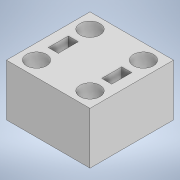
# Autodesk Inventor part: SiPM cover
Saved by Autodesk Inventor 2020 (Build 240168000, 168)
## iProperties
Created: 2021-06-25
Part Number: SiPM cover
Material: Generic
Document SubType Name: Modeling
Designer: alejandrosalazar
Density: 1 g/cm^3
Appearance: Default
Author: alejandrosalazar
Autodesk Inventor part; units mm, degrees
ref_plane "YZ Plane" through (0, 0, 0) normal (1, 0, 0) x (0, 1, 0)
ref_plane "XZ Plane" through (0, 0, 0) normal (0, 1, 0) x (-1, 0, 0)
ref_plane "XY Plane" through (0, 0, 0) normal (0, 0, 1) x (1, 0, 0)
sketch "Sketch1" plane through (0, 0, 0) normal (0, 1, 0) x (-1, 0, 0)
  line L0 (0, 0) -> (-25, 0)
  line L1 (-25, 0) -> (-25, 25)
  line L2 (-25, 25) -> (0, 25)
  line L3 (0, 25) -> (0, 0)
  line L4 (-10, 12.5) -> (-10, 15)
  line L5 (-10, 15) -> (-12.5, 15)
  line L6 (-10, 12.5) -> (-10, 10)
  line L7 (-10, 10) -> (-12.5, 10)
  line L8 (-15, 12.5) -> (-15, 15)
  line L9 (-15, 15) -> (-12.5, 15)
  line L10 (-15, 12.5) -> (-15, 10)
  line L11 (-15, 10) -> (-12.5, 10)
  circle A0 centre (-4.5, 4.5) radius 3
  circle A1 centre (-20.5, 20.5) radius 3
  circle A2 centre (-4.5, 20.5) radius 3
  circle A3 centre (-20.5, 4.5) radius 3
  dimension "d0" = 25
  dimension "d1" = 25
  dimension "d2" = 2.5
  dimension "d3" = 2.5
  dimension "d4" = 2.5
  dimension "d5" = 2.5
  dimension "d6" = 2.5
  dimension "d8" = 6
  dimension "d9" = 6
  dimension "d10" = 6
  dimension "d11" = 6
  constraints: 24 end point, 4 centre point, 3 point on line, 2 parallel, 1 horizontal, 1 perpendicular
  measures "d0" distance of L1.end L2.end
  measures "d1" distance of L0.end L1.end
  measures "d2" distance of L5.end L4.end
  measures "d3" distance of L4.end L4.start
  measures "d4" distance of L6.start L6.end
  measures "d5" distance of L8.end L9.end
  measures "d6" distance of L8.start L8.end
  measures "d8" diameter of A0
  measures "d9" diameter of A1
  measures "d10" diameter of A2
  measures "d11" diameter of A3
extrude "Extrusion1" add sketch "Sketch1" along normal blind 5
sketch "Sketch4" plane through (0, 0, 0) normal (0, -1, 0) x (1, 0, 0)
  line L0 (0, 0) -> (0, 25) projected
  line L1 (25, 25) -> (25, 0) projected
  line L2 (0, 25) -> (25, 25)
  line L3 (25, 25) -> (25, 0)
  line L4 (25, 0) -> (0, 0)
  line L5 (0, 0) -> (0, 25)
  line L6 (0.5, 24.5) -> (24.5, 24.5)
  line L7 (24.5, 24.5) -> (24.5, 0.5)
  line L8 (24.5, 0.5) -> (0.5, 0.5)
  line L9 (0.5, 0.5) -> (0.5, 24.5)
  dimension "d18" = 24
  dimension "d19" = 24
  constraints: 16 end point, 4 parallel, 2 horizontal, 2 perpendicular
  measures "d18" distance of L7.end L8.end
  measures "d19" distance of L6.end L7.end
extrude "Extrusion3" add sketch "Sketch4" along normal blind 0.5
sketch "Sketch5" plane through (0, 5, 0) normal (0, 1, 0) x (1, 0, 0)
  line L0 (20.5, -15.5) -> (17, -15.5)
  line L1 (17, -15.5) -> (17, -9.5)
  line L2 (17, -9.5) -> (20.5, -9.5)
  line L3 (20.5, -15.5) -> (24, -15.5)
  line L4 (24, -15.5) -> (24, -9.5)
  line L5 (24, -9.5) -> (20.5, -9.5)
  line L6 (8, -15.5) -> (4.5, -15.5)
  line L7 (4.5, -9.5) -> (8, -9.5)
  line L8 (8, -9.5) -> (8, -15.5)
  line L9 (4.5, -15.5) -> (1, -15.5)
  line L10 (1, -15.5) -> (1, -9.5)
  line L11 (1, -9.5) -> (4.5, -9.5)
  circle A0 centre (20.5, -20.5) radius 3
  circle A1 centre (4.5, -20.5) radius 3
  circle A2 centre (20.5, -4.5) radius 3
  circle A3 centre (4.5, -4.5) radius 3
  line L12 (15, -15) -> (10, -15) projected
  line L13 (10, -10) -> (15, -10) projected
  line L14 (15, -15) -> (10, -15)
  line L15 (10, -15) -> (10, -10)
  line L16 (10, -10) -> (15, -10)
  line L17 (15, -10) -> (15, -15)
  line L18 (25, -25) -> (0, -25) projected
  line L19 (25, -25) -> (0, -25)
  line L20 (0, -25) -> (0, 0)
  line L21 (0, 0) -> (25, 0)
  line L22 (25, 0) -> (25, -25)
  dimension "d22" = 3.5
  dimension "d23" = 6
  dimension "d24" = 3.5
  dimension "d25" = 3.5
  dimension "d26" = 6
  dimension "d27" = 3.5
  dimension "d28" = 6
  dimension "d29" = 6
  dimension "d30" = 6
  dimension "d31" = 6
  constraints: 40 end point, 8 parallel, 6 horizontal, 5 perpendicular, 4 centre point, 2 point on line
  measures "d22" distance of L1.end L2.end
  measures "d23" distance of L0.end L1.end
  measures "d24" distance of L5.end L4.end
  measures "d25" distance of L7.start L7.end
  measures "d26" distance of L6.end L7.start
  measures "d27" distance of L10.end L11.end
  measures "d28" diameter of A0
  measures "d29" diameter of A1
  measures "d30" diameter of A2
  measures "d31" diameter of A3
extrude "Extrusion4" add sketch "Sketch5" along normal blind 5
sketch "Sketch6" plane through (0, 10, 0) normal (0, 1, 0) x (1, 0, 0)
  line L0 (17, -15.5) -> (24, -15.5) projected
  line L1 (17, -9.5) -> (24, -9.5) projected
  line L2 (20.5, -15.5) -> (22, -15.5)
  line L3 (22, -15.5) -> (22, -9.5)
  line L4 (22, -9.5) -> (20.5, -9.5)
  line L5 (20.5, -15.5) -> (19, -15.5)
  line L6 (19, -15.5) -> (19, -9.5)
  line L7 (19, -9.5) -> (20.5, -9.5)
  line L8 (8, -15.5) -> (1, -15.5) projected
  line L9 (8, -9.5) -> (1, -9.5) projected
  line L10 (4.5, -15.5) -> (6, -15.5)
  line L11 (6, -15.5) -> (6, -9.5)
  line L12 (6, -9.5) -> (4.5, -9.5)
  line L13 (4.5, -15.5) -> (3, -15.5)
  line L14 (3, -15.5) -> (3, -9.5)
  line L15 (3, -9.5) -> (4.5, -9.5)
  line L16 (25, -25) -> (0, -25) projected
  line L17 (25, -25) -> (0, -25)
  line L18 (0, -25) -> (0, 0)
  line L19 (0, 0) -> (25, 0)
  line L20 (25, 0) -> (25, -25)
  circle A0 centre (4.5, -20.5) radius 3
  circle A1 centre (20.5, -20.5) radius 3
  circle A2 centre (20.5, -4.5) radius 3
  circle A3 centre (4.5, -4.5) radius 3
  dimension "d34" = 1.5
  dimension "d35" = 1.5
  dimension "d36" = 1.5
  dimension "d37" = 1.5
  dimension "d38" = 6
  dimension "d39" = 6
  dimension "d40" = 6
  dimension "d41" = 6
  constraints: 32 end point, 6 parallel, 5 horizontal, 5 perpendicular, 4 centre point, 4 point on line, 2 midpoint
  measures "d34" distance of L4.end L3.end
  measures "d35" distance of L6.end L7.end
  measures "d36" distance of L12.end L11.end
  measures "d37" distance of L14.end L15.end
  measures "d38" diameter of A0
  measures "d39" diameter of A1
  measures "d40" diameter of A2
  measures "d41" diameter of A3
extrude "Extrusion5" add sketch "Sketch6" along normal blind 5
body "Solid1"
